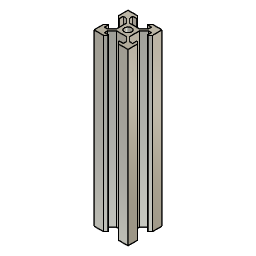
WIP Delta Build P0.01 (Autodesk Fusion 360 archive; units mm, degrees)
design "2020 Extrusion"
Autodesk Fusion 360 part; units mm, degrees
sketch "Sketch1" plane through (0, 0, 0) normal (0, 0, -1) x (1, 0, 0)
  circle A0 centre (0, 0) radius 2.1
  line L0 (5.5, 8.3) -> (5.5, 6.5607)
  line L1 (5.5, 6.5607) -> (2.8393, 3.9)
  line L2 (2.8393, 3.9) -> (-2.8393, 3.9)
  line L3 (-2.8393, 3.9) -> (-5.5, 6.5607)
  line L4 (-5.5, 6.5607) -> (-5.5, 8.3)
  line L5 (-5.5, 8.3) -> (-3.1, 8.3)
  line L6 (-3.1, 8.3) -> (-3.1, 8.7128)
  line L7 (-3.1, 8.7128) -> (-4.386, 10)
  line L8 (-4.386, 10) -> (-10, 10)
  line L9 (-10, 10) -> (-10, 4.386)
  line L10 (-10, 4.386) -> (-8.7128, 3.1)
  line L11 (-8.7128, 3.1) -> (-8.3, 3.1)
  line L12 (-8.3, 3.1) -> (-8.3, 5.5)
  line L13 (-8.3, 5.5) -> (-6.5607, 5.5)
  line L14 (-6.5607, 5.5) -> (-3.9, 2.8393)
  line L15 (-3.9, 2.8393) -> (-3.9, -2.8393)
  line L16 (-3.9, -2.8393) -> (-6.5607, -5.5)
  line L17 (-6.5607, -5.5) -> (-8.3, -5.5)
  line L18 (-8.3, -5.5) -> (-8.3, -3.1)
  line L19 (-8.3, -3.1) -> (-8.7128, -3.1)
  line L20 (-8.7128, -3.1) -> (-10, -4.386)
  line L21 (-10, -4.386) -> (-10, -10)
  line L22 (-10, -10) -> (-4.386, -10)
  line L23 (-4.386, -10) -> (-3.1, -8.7128)
  line L24 (-3.1, -8.7128) -> (-3.1, -8.3)
  line L25 (-3.1, -8.3) -> (-5.5, -8.3)
  line L26 (-5.5, -8.3) -> (-5.5, -6.5607)
  line L27 (-5.5, -6.5607) -> (-2.8393, -3.9)
  line L28 (-2.8393, -3.9) -> (2.8393, -3.9)
  line L29 (2.8393, -3.9) -> (5.5, -6.5607)
  line L30 (5.5, -6.5607) -> (5.5, -8.3)
  line L31 (5.5, -8.3) -> (3.1, -8.3)
  line L32 (3.1, -8.3) -> (3.1, -8.7128)
  line L33 (3.1, -8.7128) -> (4.386, -10)
  line L34 (4.386, -10) -> (10, -10)
  line L35 (10, -10) -> (10, -4.386)
  line L36 (10, -4.386) -> (8.7128, -3.1)
  line L37 (8.7128, -3.1) -> (8.3, -3.1)
  line L38 (8.3, -3.1) -> (8.3, -5.5)
  line L39 (8.3, -5.5) -> (6.5607, -5.5)
  line L40 (6.5607, -5.5) -> (3.9, -2.8393)
  line L41 (3.9, -2.8393) -> (3.9, 2.8393)
  line L42 (3.9, 2.8393) -> (6.5607, 5.5)
  line L43 (6.5607, 5.5) -> (8.3, 5.5)
  line L44 (8.3, 5.5) -> (8.3, 3.1)
  line L45 (8.3, 3.1) -> (8.7128, 3.1)
  line L46 (8.7128, 3.1) -> (10, 4.386)
  line L47 (10, 4.386) -> (10, 10)
  line L48 (10, 10) -> (4.386, 10)
  line L49 (4.386, 10) -> (3.1, 8.7128)
  line L50 (3.1, 8.7128) -> (3.1, 8.3)
  line L51 (3.1, 8.3) -> (5.5, 8.3)
sketch "Sketch2" plane through (0, 0, 0) normal (0, 0, 1) x (1, 0, 0)
sketch "Sketch3" plane through (0, 0, 0) normal (0, 0, 1) x (1, 0, 0)
extrude "Extrude1" add sketch "Sketch1" along normal blind 100
move_body "Move1" bodies 1 to x (1, 0, 0) y (0, 1, 0) z (0, 0, 1) at (45, 0, 0)
move_body "Align1" bodies 1 to x (1, 0, 0) y (0, 1, 0) z (0, 0, 1) at (-45, 0, 100)
equation "Length = 100 mm"
equation "d2 = Length"

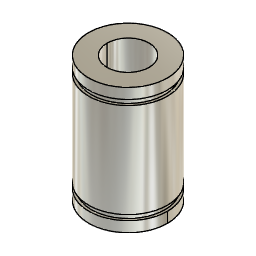
design "LM8UU"
Autodesk Fusion 360 part; units mm, degrees
sketch "Sketch1" plane through (0, 0, 15) normal (0, 0, 1) x (-1, 0, 0)
  circle A0 centre (-120.2406, -9.8454) radius 4
  circle A1 centre (-120.2406, -9.8454) radius 7.5
  circle A2 centre (-120.2406, -9.8161) radius 4
  circle A3 centre (-120.2406, -9.8161) radius 4
  circle A4 centre (-120.2406, -9.8161) radius 7.5
  dimension "d338_1" = 15
  constraint concentric A2 A3
  constraint concentric A2 A4
  measures "d338_1" diameter of A4
extrude "Extrude1" add sketch "Sketch1" along normal blind 2 contours A1 A4 picked at (-113.9366, -10.2172)
sketch "Sketch2" plane through (0, 0, 17) normal (0, 0, 1) x (-1, 0, 0)
  arc A0 (-116.2406, -9.8307) -> (-124.2406, -9.8307) centre (-120.2406, -9.8161) ccw
  arc A1 (-124.2406, -9.8307) -> (-116.2406, -9.8307) centre (-120.2406, -9.8454) ccw
  arc A2 (-112.7406, -9.8307) -> (-127.7406, -9.8307) centre (-120.2406, -9.8454) ccw
  arc A3 (-127.7406, -9.8307) -> (-112.7406, -9.8307) centre (-120.2406, -9.8161) ccw
  arc A4 (-127.7406, -9.8307) -> (-112.7406, -9.8307) centre (-120.2406, -9.8161) ccw
  arc A5 (-112.7406, -9.8307) -> (-127.7406, -9.8307) centre (-120.2406, -9.8454) ccw
  circle A6 centre (-120.2406, -9.8161) radius 4
  circle A7 centre (-120.2406, -9.8454) radius 7
  point P0 (-127.7406, -9.8307)
  dimension "d341_1" = 14
  constraint concentric A1 A7
  measures "d341_1" diameter of A7
extrude "Extrude2" add sketch "Sketch2" along normal blind 1 contours A7
sketch "Sketch3" plane through (0, 0, 18) normal (0, 0, 1) x (-1, 0, 0)
  arc A0 (-116.2406, -9.8307) -> (-124.2406, -9.8307) centre (-120.2406, -9.8161) ccw
  arc A1 (-124.2406, -9.8307) -> (-116.2406, -9.8307) centre (-120.2406, -9.8454) ccw
  circle A2 centre (-120.2406, -9.8161) radius 4
  circle A3 centre (-120.2406, -9.8161) radius 7.5
  dimension "d344_1" = 15
  constraint concentric A2 A3
  measures "d344_1" diameter of A3
extrude "Extrude3" add sketch "Sketch3" along normal blind 21
sketch "Sketch4" plane through (0, 0, 39) normal (0, 0, 1) x (-1, 0, 0)
  arc A0 (-116.2406, -9.8307) -> (-124.2406, -9.8307) centre (-120.2406, -9.8161) ccw
  arc A1 (-124.2406, -9.8307) -> (-116.2406, -9.8307) centre (-120.2406, -9.8454) ccw
  circle A2 centre (-120.2406, -9.8161) radius 7.5
  circle A3 centre (-120.2406, -9.8161) radius 4
  circle A4 centre (-120.2406, -9.8161) radius 7
  dimension "d347_1" = 14
  constraint concentric A3 A4
  measures "d347_1" diameter of A4
extrude "Extrude4" add sketch "Sketch4" along normal blind 1 contours A4
sketch "Sketch5" plane through (0, 0, 40) normal (0, 0, 1) x (-1, 0, 0)
  arc A0 (-116.2406, -9.8307) -> (-124.2406, -9.8307) centre (-120.2406, -9.8161) ccw
  arc A1 (-124.2406, -9.8307) -> (-116.2406, -9.8307) centre (-120.2406, -9.8454) ccw
  circle A2 centre (-120.2406, -9.8161) radius 7
  circle A3 centre (-120.2406, -9.8161) radius 4
  circle A4 centre (-120.2406, -9.8161) radius 7.5
  dimension "d350_1" = 15
  constraint concentric A3 A4
  measures "d350_1" diameter of A4
extrude "Extrude5" add sketch "Sketch5" along normal blind 2 contours A2 | A4
extrude "Extrude6" cut 1 faces at (126.546, 10.1936, 42) along direction (0, 0, -1) blind 3
sketch "Sketch6" plane through (120.2406, 9.8161, 37) normal (0, 0, 1) x (1, 0, 0)
move_body "Align1" bodies 1 to x (1, 0, 0) y (0, 1, 0) z (0, 0, 1) at (-120.2406, -9.8161, -15)
ref_plane "WorkPlane2" through (0, 0, 22) normal (0, 0, 1) x (-1, 0, 0)
sketch "Sketch7" plane through (0, 0, 22) normal (0, 0, 1) x (1, 0, 0)
  circle A0 centre (0, 0) radius 7
  circle A1 centre (0, 0) radius 7.5
  dimension "d5" = 14
  dimension "d6" = 15
  constraint coincident A0.centre A1.centre
  measures "d5" diameter of A0
  measures "d6" diameter of A1
extrude "Extrude7" cut sketch "Sketch7" against normal blind 1

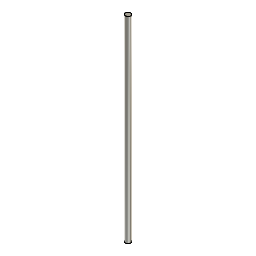
design "Linear Rod"
Autodesk Fusion 360 part; units mm, degrees
sketch "Sketch1" plane through (0, 0, 0) normal (0, 0, 1) x (1, 0, 0)
  circle A0 centre (0, 0) radius 4
  dimension "d3" = 8
  constraint coincident A0.centre origin
  measures "d3" diameter of A0
extrude "Extrude1" add sketch "Sketch1" along normal blind 300
equation "Circumference = 8 mm"
equation "Length = 300 mm"
equation "d3 = Circumference"
equation "d4 = Length"

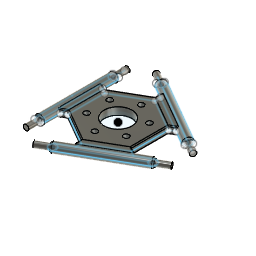
design "Effector"
Autodesk Fusion 360 part; units mm, degrees
sketch "Sketch1" plane through (0, 0, 0) normal (0, 0, 1) x (1, 0, 0)
  line L0 (0, 20) -> (-17.3205, 10)
  line L1 (-17.3205, 10) -> (-17.3205, -10)
  line L2 (-17.3205, -10) -> (0, -20)
  line L3 (0, -20) -> (17.3205, -10)
  line L4 (17.3205, -10) -> (17.3205, 10)
  line L5 (17.3205, 10) -> (0, 20)
  line L6 (-7.3205, -27.3205) -> (27.3205, -7.3205)
  line L7 (12.5, -21.6506) -> (29.8205, -11.6506)
  line L8 (12.5, -21.6506) -> (-4.8205, -31.6506)
  line L9 (0, -20) -> (0, -23.094)
  line L10 (17.3205, -10) -> (20, -11.547)
  circle A0 centre (-6.0705, -29.4856) radius 2
  circle A1 centre (28.5705, -9.4856) radius 2
  line L11 (-4.8205, -31.6506) -> (-6.3097, -31.4712)
  line L12 (-7.3205, -27.3205) -> (-7.9097, -28.6999)
  line L13 (27.3205, -7.3205) -> (28.8097, -7.4999)
  line L14 (29.8205, -11.6506) -> (30.4097, -10.2712)
  line L15 (-25, 0) -> (-25, -20)
  line L16 (-25, 0) -> (-25, 20)
  circle A2 centre (-22.5, -20) radius 2
  line L17 (-25, -20) -> (-24.1, -21.2)
  line L18 (-20, -20) -> (-20.9, -21.2)
  line L19 (-20, -20) -> (-20, 20)
  line L20 (-17.3205, -10) -> (-20, -11.547)
  line L21 (-17.3205, 10) -> (-20, 11.547)
  circle A3 centre (-22.5, 20) radius 2
  line L22 (-20, 20) -> (-20.9, 21.2)
  line L23 (-25, 20) -> (-24.1, 21.2)
  line L24 (12.5, 21.6506) -> (-4.8205, 31.6506)
  line L25 (29.8205, 11.6506) -> (30.4097, 10.2712)
  line L26 (12.5, 21.6506) -> (29.8205, 11.6506)
  line L27 (-4.8205, 31.6506) -> (-6.3097, 31.4712)
  circle A4 centre (-6.0705, 29.4856) radius 2
  line L28 (-7.3205, 27.3205) -> (27.3205, 7.3205)
  line L29 (-7.3205, 27.3205) -> (-7.9097, 28.6999)
  line L30 (27.3205, 7.3205) -> (28.8097, 7.4999)
  circle A5 centre (28.5705, 9.4856) radius 2
  line L31 (0, 20) -> (0, 23.094)
  line L32 (17.3205, 10) -> (20, 11.547)
  line L33 (-22.5, -20) -> (-22.5, 20)
  line L34 (-22.5, 20) -> (-22.5, 26)
  line L35 (28.5705, -9.4856) -> (-6.0705, -29.4856)
  line L36 (28.5705, 9.4856) -> (-6.0705, 29.4856)
  line L37 (-6.0705, 29.4856) -> (-10.3312, 31.9455)
  line L38 (-10.3312, 31.9455) -> (33.559, 6.6054)
  dimension "d19" = 4
  constraint coincident L6 L9.end
  constraint vertical L9
  constraint coincident L6 L10.end
  constraint coincident A0 L11.end
  constraint tangent A0 L11
  constraint coincident A0 L12.end
  constraint tangent A0 L12
  constraint coincident A1 L13.end
  constraint tangent A1 L13
  constraint parallel L11 L13
  constraint coincident A1 L14.end
  constraint tangent A1 L14
  constraint coincident A2.centre L33.start
  constraint coincident A3.centre L33.end
  constraint vertical L33
  constraint parallel L33 L34
  constraint coincident A1.centre L35.start
  constraint coincident A0.centre L35.end
  constraint coincident A5.centre L36.start
  constraint coincident A4.centre L36.end
  constraint parallel L28 L36
  constraint parallel L28 L37
  constraint parallel L36 L38
  measures "d19" diameter of A0
revolve "Revolve1" add sketch "Sketch1" angle 360 about axis through (-22.5, -20, 0) along (0, 1, 0) contours A2 L18 L19 A3 L22 L33 | A3 L33 L34 | A2 picked at (-21.1735, 19.9051) makes body 1
sketch "Sketch2" plane through (0, 0, 0) normal (0, 1, 0) x (1, 0, 0)
  circle A0 centre (-22.5, 0) radius 2.5
  circle A1 centre (-22.5, 0) radius 1.5
  dimension "d23" = 3
  constraint concentric A0 A1
  measures "d23" diameter of A1
extrude "Extrude1" cut sketch "Sketch2" along normal mid plane 45 contours A1 bodies 1
fillet "Fillet1" radius 0.25 1 edges at (-23.8985, -21.3229, 0.5424) on bodies 1
fillet "Fillet2" radius 0.25 1 edges at (-23.8985, 21.3229, -0.5424) on bodies 1
extrude "Extrude2" add sketch "Sketch1" along normal mid plane 4 separate body contours L1 L19 L20 L21 makes body 2
extrude "Extrude3" add 1 faces at (-20, -3.849, -0.6667) along direction (-1, 0, 0) blind 1 on bodies 2 bodies 1 2
fillet "Fillet3" radius 0.5 4 edges at (-18.6603, 10.7735, -2) (-20.5, 11.547, -2) (-18.6603, 10.7735, 2) (-20.5, 11.547, 2) on bodies 1
fillet "Fillet4" radius 0.5 4 edges at (-18.6603, -10.7735, -2) (-18.6603, -10.7735, 2) (-20.5, -11.547, 2) (-20.5, -11.547, -2) on bodies 1
move_body "Move1" bodies 1 to x (-0.5, -0.866025, 0) y (0.866025, -0.5, 0) z (0, 0, 1) at (0, 0, 0)
mirror "Mirror1" about plane through (0, 0, 0) normal (0, 1, 0) of bodies 1 makes body 3
move_body "Move2" bodies 3 to x (-0.5, -0.866025, 0) y (0.866025, -0.5, 0) z (0, 0, 1) at (0, 0, 0)
mirror "Mirror2" about plane through (0, 0, 0) normal (0, 1, 0) of bodies 1 makes body 4
extrude "Extrude4" add sketch "Sketch1" along normal mid plane 4 separate body contours L0 L1 L2 L3 L4 L5 makes body 5
fillet "Fillet5" radius 0.5 1 edges at (17.3205, 0, -2) on bodies 5
fillet "Fillet6" radius 0.5 1 edges at (17.3205, 0, 2) on bodies 5
fillet "Fillet7" radius 0.5 3 edges at (-8.6603, -15, 2) (-8.6603, 15, -2) (-8.6603, -15, -2) on bodies 5
fillet "Fillet8" radius 0.5 1 edges at (-8.6603, 15, 2) on bodies 5
sketch "Sketch3" plane through (0, 0, 2) normal (0, 0, 1) x (-1, 0, 0)
  line L0 (-0.5, -19.7113) -> (17.3205, -9.4226)
  line L1 (17.3205, -9.4226) -> (17.3205, 9.4226)
  line L2 (17.3205, 9.4226) -> (-0.5, 19.7113)
  line L3 (-0.5, 19.7113) -> (-16.8205, 10.2887)
  line L4 (-16.8205, 10.2887) -> (-16.8205, -10.2887)
  line L5 (-16.8205, -10.2887) -> (-0.5, -19.7113)
  circle A0 centre (0, 0) radius 12.5
  circle A1 centre (0.0762, 12.4998) radius 1.5
  circle A2 centre (-10.787, 6.3159) radius 1.5
  circle A3 centre (-10.8632, -6.1839) radius 1.5
  circle A4 centre (-0.0762, -12.4998) radius 1.5
  circle A5 centre (10.787, -6.3159) radius 1.5
  circle A6 centre (10.8632, 6.1839) radius 1.5
  circle A7 centre (0, 0) radius 7.5
  dimension "d54" = 25
  dimension "d55" = 3
  dimension "d57" = 360
  dimension "d58" = 15
  constraint coincident A0.centre A7.centre
  constraint coincident A0 A1.centre
  measures "d54" diameter of A0
  measures "d55" diameter of A1
  measures "d58" diameter of A7
extrude "Extrude5" cut sketch "Sketch3" against normal blind 14 contours A0 A6 | A0 A6 | A0 A5 | A0 A5 | A0 A1 | A0 A1 | A0 A4 | A0 A4 | A0 A2 | A0 A2 | A0 A3 | A0 A3 | A7 bodies 5
sketch "Sketch4" plane through (0, 0, 0) normal (0, 0, 1) x (1, 0, 0)
  circle A0 centre (0, 0) radius 1.5
  dimension "d61" = 3
  constraint coincident A0.centre origin
  measures "d61" diameter of A0
extrude "Extrude6" add sketch "Sketch4" along normal blind 55 separate body makes body 6
move_body "Align1" bodies 6 to x (-0.5, 0.866025, 0) y (0, 0, -1) z (-0.866025, -0.5, 0) at (35.0657, -5.7356, 0)
copy_body "CopyPasteBodies1" bodies 6 makes body 7
move_body "Move3" bodies 7 to x (1, 0, 0) y (0, 1, 0) z (0, 0, 1) at (55.4256, 32, 0)
mirror "Mirror3" about plane through (0, 0, 0) normal (0, 1, 0) of bodies 6 makes body 8
move_body "Align2" bodies 7 to x (-0.5, -0.866025, 0) y (0.866025, -0.5, 0) z (0, 0, 1) at (0, 64, 0)
